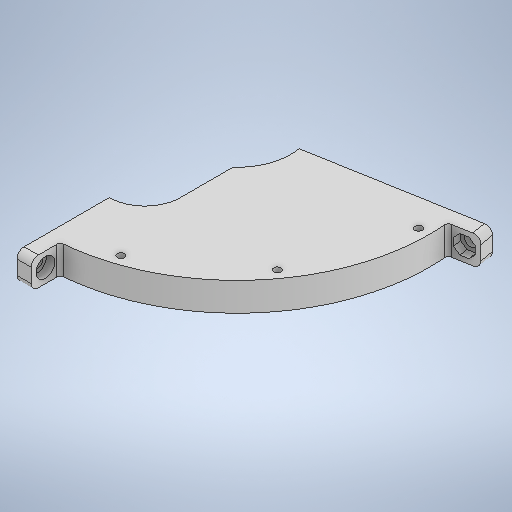
# Autodesk Inventor part: Cylinder Spacer Top_Q3
Saved by Autodesk Inventor 2025 (Build 290162000, 162)
## iProperties
Created: 2024-04-28
Part Number: Cylinder Spacer Top_Q3
Material: Generic
Document SubType Name: Modeling
Designer: Thienan Hoang
Density: 1 g/cm^3
Appearance: Default
Author: Thienan Hoang
Autodesk Inventor part; units mm, degrees
ref_plane "YZ Plane" through (0, 0, 0) normal (1, 0, 0) x (0, 1, 0)
ref_plane "XZ Plane" through (0, 0, 0) normal (0, 1, 0) x (-1, 0, 0)
ref_plane "XY Plane" through (0, 0, 0) normal (0, 0, 1) x (1, 0, 0)
sketch "Sketch1" plane through (0, 0, 0) normal (0, 1, 0) x (-1, 0, 0)
  circle A0 centre (0, 0) radius 135
  circle A1 centre (0, 0) radius 110
  dimension "d0" = 270
  dimension "d1" = 220
  constraints: 2 centre point, 2 coincident
  measures "d0" diameter of A0
  measures "d1" diameter of A1
extrude "Extrusion1" add sketch "Sketch1" along normal blind 55
sketch "Sketch2" plane through (0, 0, 0) normal (0, 0, 1) x (1, 0, 0)
  circle A0 centre (0, 5) radius 18
  line L0 (135, 0) -> (-135, 0) projected
  point P0 (0, 0)
  dimension "d4" = 36
  dimension "d5" = 5
  constraints: 1 centre point
  measures "d4" diameter of A0
  measures "d5" distance from line of L0 A0.centre
extrude "Extrusion2" cut sketch "Sketch2" against normal through all
sketch "Sketch3" plane through (0, 0, 0) normal (0, -1, 0) x (1, 0, 0)
  circle A0 centre (0, 0) radius 140
  constraints: 1 centre point, 1 coincident
extrude "Extrusion3" cut sketch "Sketch3" against normal blind 20
sketch "Sketch4" plane through (0, 20, 0) normal (0, -1, 0) x (1, 0, 0)
  line L0 (0, 0) -> (70, 0)
  line L1 (80, -100) -> (60, -100)
  line L2 (60, -100) -> (60, 100)
  line L3 (60, 100) -> (80, 100)
  line L4 (80, 100) -> (80, -100)
  line L5 (80, -100) -> (60, 100) construction
  line L6 (60, -100) -> (80, 100) construction
  dimension "d10" = 70
  dimension "d11" = 20
  dimension "d12" = 200
  constraints: 14 end point, 2 horizontal, 2 midpoint, 2 parallel, 1 perpendicular
  measures "d10" distance of L0.start L0.end
  measures "d11" distance of L2.end L3.end
  measures "d12" distance of L1.end L2.end
extrude "Extrusion4" cut sketch "Sketch4" against normal through all
sketch "Sketch5" plane through (0, 55, 0) normal (0, 1, 0) x (1, 0, 0)
  circle A0 centre (0, 0) radius 127.5
  circle A1 centre (127.5, 0) radius 2
  circle A2 centre (103.1497, 74.9426) radius 2
  circle A3 centre (39.3997, 121.2597) radius 2
  circle A4 centre (-39.3997, 121.2597) radius 2
  circle A5 centre (-103.1497, 74.9426) radius 2
  circle A6 centre (-127.5, 0) radius 2
  circle A7 centre (-103.1497, -74.9426) radius 2
  circle A8 centre (-39.3997, -121.2597) radius 2
  circle A9 centre (39.3997, -121.2597) radius 2
  circle A10 centre (103.1497, -74.9426) radius 2
  dimension "d15" = 255
  dimension "d16" = 4
  dimension "d19" = 360
  constraints: 10 centre point, 1 coincident, 1 horizontal alignment, 23 other
  measures "d16" diameter of A1
hole "Hole1" at (127.5, 55, 0) at (103.1497, 55, 74.9426) at (39.3997, 55, 121.2597) at (-39.3997, 55, 121.2597) at (-103.1497, 55, 74.9426) at (-127.5, 55, 0) at (-103.1497, 55, -74.9426) at (-39.3997, 55, -121.2597) at (39.3997, 55, -121.2597) at (103.1497, 55, -74.9426) direction (0, -1, 0) diameter 5 end through all
sketch "Sketch6" plane through (0, 55, 0) normal (0, 1, 0) x (1, 0, 0)
  circle A0 centre (0, 0) radius 140
  constraints: 1 centre point, 1 coincident
extrude "Extrusion5" cut sketch "Sketch6" against normal blind 15
sketch "Sketch7" plane through (0, 40, 0) normal (0, 1, 0) x (1, 0, 0)
  circle A0 centre (0, 0) radius 140
  line L0 (80, -100) -> (80, -75.4983) projected
  line L1 (80, -100) -> (80, -75.4983)
  line L2 (60, -100) -> (80, -100) projected
  line L3 (80, -100) -> (60, -100)
  line L4 (60, -100) -> (60, -92.1954)
  line L5 (60, 100) -> (60, 92.1954) projected
  line L6 (60, 92.1954) -> (60, 100)
  line L7 (60, 100) -> (80, 100)
  line L8 (80, 100) -> (80, 75.4983)
  arc A1 (80, -75.4983) -> (80, 75.4983) centre (0, 0) ccw
  arc A2 (60, 92.1954) -> (60, -92.1954) centre (0, 0) ccw
  arc A3 (-25, -65) -> (25, -65) centre (0, -65) ccw
  arc A4 (25, 65) -> (-25, 65) centre (0, 65) ccw
  arc A5 (25, -27.9508) -> (25, 27.9508) centre (0, 0) ccw
  arc A6 (-25, 27.9508) -> (-25, -27.9508) centre (0, 0) ccw
  line L9 (25, 65) -> (25, 27.9508)
  line L10 (25, -27.9508) -> (25, -65)
  line L11 (-25, -65) -> (-25, -27.9508)
  line L12 (-25, 27.9508) -> (-25, 65)
  constraints: 20 end point, 12 point on circle, 7 centre point, 7 equal length, 3 perpendicular, 2 coincident
extrude "Extrusion6" add sketch "Sketch7" against normal blind 1 contours L2 L4 A2 L5 L7 L8 A1 L0
sketch "Sketch8" plane through (0, 39, 0) normal (0, -1, 0) x (1, 0, 0)
  line L0 (80, -75.4983) -> (80, -100) projected
  line L1 (80, -100) -> (60, -100)
  line L2 (60, -100) -> (60, 100)
  line L3 (60, 100) -> (80, 100)
  line L4 (80, 100) -> (80, 75.4983)
  line L5 (80, -75.4983) -> (80, -100)
  arc A0 (80, -75.4983) -> (80, 75.4983) centre (0, 0) ccw
  arc A1 (60, 92.1954) -> (60, -92.1954) centre (0, 0) ccw
  constraints: 10 end point, 4 point on circle, 3 parallel, 2 centre point, 2 point on line, 1 coincident, 1 horizontal, 1 perpendicular
extrude "Extrusion7" add sketch "Sketch8" along normal blind 14 contours L0 L1 L2 L3 L4 A0
sketch "Sketch9" plane through (0, 20, 0) normal (0, -1, 0) x (1, 0, 0)
  arc A0 (9.9499, -134.6328) -> (-9.9499, -134.6328) centre (0, 0) ccw projected
  spline S0 degree 7 poles (9.9499, -134.6328) (9.4556, -134.6694) (8.9421, -134.7052) (8.4096, -134.74) (7.8582, -134.7735) (7.2882, -134.8052) (6.6998, -134.835) (5.2633, -134.8999) (4.3998, -134.933) (3.5087, -134.9604) (2.5962, -134.9814) (1.6691, -134.9951) (0.7345, -135.0012) (-1.7136, -134.9976) (-3.2083, -134.9756) (-4.6621, -134.9347) (-6.0536, -134.8776) (-7.364, -134.8084) (-8.5782, -134.7318) (-9.7236, -134.6494) (-9.7616, -134.6466) (-9.7995, -134.6439) (-9.8372, -134.6411) (-9.8749, -134.6384) (-9.9124, -134.6356) (-9.9499, -134.6328) knots 0 0 0 0 0 0 0 0 0.214533 0.214533 0.214533 0.214533 0.214533 0.214533 0.508291 0.508291 0.508291 0.508291 0.508291 0.508291 0.983641 0.983641 0.983641 0.983641 0.983641 0.983641 1 1 1 1 1 1 1 1 projected
  line L0 (0, 135) -> (0, -135)
  line L1 (132.949, -23.4425) -> (-132.949, 23.4425)
  point P0 (0, 0)
  dimension "d40" = 80
  constraints: 4 end point, 3 point on circle, 2 midpoint, 1 line through centre, 1 vertical, 2 other
  measures "d40" angle of L0 L1
extrude "Extrusion8" cut sketch "Sketch9" against normal through all contours S0 L0 L1 A0 | S0 A0 L1 L0 | L0 L1 A0 picked at (-5.2242, 89.6957)
sketch "Sketch10" plane through (0, 20, 110) normal (-1, 0, 0) x (0, 0, 1)
  line L0 (25, 0) -> (-133.4425, 0) projected
  line L1 (22.5, 0) -> (40, 0)
  line L2 (45, 5) -> (45, 15)
  line L3 (40, 20) -> (22.5, 20)
  line L4 (22.5, 20) -> (22.5, 0)
  line L5 (25, 20) -> (25, 0) projected
  arc A0 (40, 0) -> (45, 5) centre (40, 5) ccw
  arc A1 (45, 15) -> (40, 20) centre (40, 15) ccw
  point P0 (-110, -20)
  point P1 (45, 20)
  point P2 (45, 0)
  dimension "d43" = 22.5
  dimension "d44" = 20
  dimension "d45" = 20
  dimension "d46" = 5
  constraints: 8 end point, 5 point on line, 4 point on circle, 4 tangent, 2 centre point, 2 parallel, 1 equal radius, 1 horizontal, 1 perpendicular
  measures "d43" distance of L3.end point (45, 20)
  measures "d44" distance of point (45, 20) point (45, 0)
  measures "d45" distance between parallel lines of L5 L2
  measures "d46" radius of A0
extrude "Extrusion9" add sketch "Sketch10" against normal blind 10
sketch "Sketch11" plane through (132.949, 20, -23.4425) normal (-0.1736482, 0, -0.9848078) x (-0.9848078, 0, 0.1736482)
  line L0 (0, 20) -> (97.5, 20) projected
  line L1 (2.5, 20) -> (-15, 20)
  line L2 (-20, 15) -> (-20, 5)
  line L3 (-15, 0) -> (2.5, 0)
  line L4 (2.5, 0) -> (2.5, 20)
  line L5 (0, 0) -> (0, 20) projected
  arc A0 (-20, 5) -> (-15, 0) centre (-15, 5) ccw
  arc A1 (-15, 20) -> (-20, 15) centre (-15, 15) ccw
  point P0 (135, -20)
  point P1 (-20, 0)
  point P2 (-20, 20)
  dimension "d49" = 22.5
  dimension "d50" = 20
  dimension "d51" = 20
  dimension "d52" = 5
  constraints: 8 end point, 5 point on line, 4 point on circle, 4 tangent, 2 centre point, 2 parallel, 1 equal radius, 1 horizontal, 1 perpendicular
  measures "d49" distance of L3.end point (-20, 0)
  measures "d50" distance of point (-20, 0) point (-20, 20)
  measures "d51" distance between parallel lines of L2 L5
  measures "d52" radius of A0
extrude "Extrusion10" add sketch "Sketch11" against normal blind 10
fillet "Fillet1" radius 2.5 2 edges at (10, 30, 134.6291) (134.3203, 30, -13.53)
sketch "Sketch12" plane through (10, 20, 110) normal (1, 0, 0) x (0, 0, -1)
  line L0 (-40, 0) -> (-26.9306, 0) projected
  line L1 (-45, 15) -> (-45, 5) projected
  point P0 (110, -20)
  point P1 (-35, 10)
  dimension "d56" = 10
  dimension "d57" = 10
  measures "d56" distance from line of L0 point (-35, 10)
  measures "d57" distance from line of L1 point (-35, 10)
hole "Hole2" at (10, 30, 145) direction (-1, 0, 0) diameter 8.2 end through all counterbore diameter 13.2 counterbore depth 6
sketch "Sketch13" plane through (134.6855, 20, -13.5944) normal (0.1736482, 0, 0.9848078) x (0.9848078, 0, -0.1736482)
  line L0 (16.6, 7.2662) -> (12.7338, 3.4)
  line L1 (12.7338, 3.4) -> (7.2662, 3.4)
  line L2 (7.2662, 3.4) -> (3.4, 7.2662)
  line L3 (3.4, 7.2662) -> (3.4, 12.7338)
  line L4 (3.4, 12.7338) -> (7.2662, 16.6)
  line L5 (7.2662, 16.6) -> (12.7338, 16.6)
  line L6 (12.7338, 16.6) -> (16.6, 12.7338)
  line L7 (16.6, 12.7338) -> (16.6, 7.2662)
  line L8 (20, 5) -> (20, 15) projected
  line L9 (1.9306, 0) -> (15, 0) projected
  point P0 (-135, -20)
  point P1 (10, 10)
  point P2 (20, 10)
  dimension "d65" = 10
  dimension "d66" = 10
  dimension "d67" = 13.2
  constraints: 16 end point, 1 midpoint, 1 vertical, 17 other
  measures "d65" distance of point (20, 10) point (10, 10)
  measures "d66" distance from line of L9 point (10, 10)
  measures "d67" distance between parallel lines of L3 L7
extrude "Extrusion11" cut sketch "Sketch13" against normal blind 6
sketch "Sketch14" plane through (133.6436, 20, -19.5033) normal (0.1736482, 0, 0.9848078) x (0.9848078, 0, -0.1736482)
  line L0 (1.9306, 0) -> (15, 0) projected
  line L1 (20, 5) -> (20, 15) projected
  point P0 (-135, -20)
  point P1 (10, 10)
  dimension "d70" = 10
  dimension "d71" = 10
  measures "d70" distance from line of L0 point (10, 10)
  measures "d71" distance from line of L1 point (10, 10)
hole "Hole3" at (143.4917, 30, -21.2398) direction (-0.1736482, 0, -0.9848078) diameter 8.2 end through all
body "Solid1"
